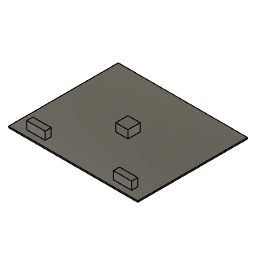
Food_Chain_Magnate_Cover v2 (Autodesk Fusion 360 design; units mm, degrees)
Autodesk Fusion 360 part; units mm, degrees
sketch "Sketch1" plane through (0, 0, 0) normal (0, 0, 1) x (1, 0, 0)
  line L0 (-25, 25) -> (187, 25)
  line L1 (187, 25) -> (187, -155)
  line L2 (187, -155) -> (-25, -155)
  line L3 (-25, -155) -> (-25, 25)
  dimension "d1" = 212
  dimension "d2" = 180
  constraint horizontal L0
  constraint vertical L1
  constraint horizontal L2
  constraint vertical L3
  measures "d1" distance of L0.start L0.end
  measures "d2" distance of L0.start L2.end
extrude "Extrude1" add sketch "Sketch1" along normal blind 2
sketch "Sketch2" plane through (0, 0, 2) normal (0, 0, 1) x (-1, 0, 0)
  line L0 (25, 155) -> (-187, 155)
  line L1 (-187, 155) -> (-187, -25)
  line L2 (-187, -25) -> (25, -25)
  line L3 (25, -25) -> (25, 155)
  line L4 (25, -25) -> (-187, 155) construction
  line L5 (25, 155) -> (-187, -25) construction
  line L6 (25, 65) -> (-81, 65) construction
  line L7 (-187, 65) -> (-81, 65) construction
  line L8 (-81, 65) -> (-81, -25) construction
  line L9 (-81, 65) -> (-81, 155) construction
  line L10 (25, 155) -> (5, 155) construction
  line L11 (5, 155) -> (5, 135) construction
  line L12 (5, 135) -> (25, 135) construction
  line L13 (25, 135) -> (25, 155) construction
  line L14 (-187, 155) -> (-167, 155) construction
  line L15 (-167, 145) -> (-167, 135)
  line L16 (-167, 135) -> (-187, 135) construction
  line L17 (-187, 135) -> (-187, 155) construction
  line L18 (-187, -25) -> (-167, -25) construction
  line L19 (-167, -25) -> (-167, -5) construction
  line L20 (-167, -5) -> (-187, -5) construction
  line L21 (-187, -5) -> (-187, -25) construction
  line L22 (25, -25) -> (5, -25) construction
  line L23 (5, -25) -> (5, -5) construction
  line L24 (5, -5) -> (25, -5) construction
  line L25 (25, -5) -> (25, -25) construction
  line L26 (-167, 135) -> (-137, 135)
  line L27 (-137, 135) -> (-137, 145)
  line L28 (-137, 145) -> (-167, 145)
  line L29 (-167, 145) -> (-167, 135) construction
  line L30 (5, 135) -> (-25, 135)
  line L31 (-25, 135) -> (-25, 145)
  line L32 (-25, 145) -> (5, 145)
  line L33 (5, 145) -> (5, 135)
  line L34 (-167, 155) -> (-167, 145) construction
  line L35 (-71, 55) -> (-91, 55)
  line L36 (-91, 55) -> (-91, 75)
  line L37 (-91, 75) -> (-71, 75)
  line L38 (-71, 75) -> (-71, 55)
  line L39 (-71, 55) -> (-91, 75) construction
  line L40 (-91, 55) -> (-71, 75) construction
  point P0 (-81, 65)
  dimension "d5" = 20
  dimension "d6" = 20
  dimension "d7" = 20
  dimension "d8" = 20
  dimension "d9" = 20
  dimension "d10" = 20
  dimension "d11" = 20
  dimension "d12" = 20
  dimension "d13" = 30
  dimension "d14" = 10
  dimension "d15" = 30
  dimension "d16" = 10
  dimension "d17" = 20
  dimension "d18" = 20
  constraint coincident L2.end L3.start
  constraint coincident L0.end L1.start
  constraint coincident L0.start L3.end
  constraint coincident L1.end L2.start
  constraint midpoint L3 L6.start
  constraint midpoint L5 P0
  constraint midpoint L1 L7.start
  constraint midpoint L2 L8.end
  constraint midpoint L0 L9.end
  constraint horizontal L10
  constraint vertical L11
  constraint horizontal L12
  constraint vertical L13
  constraint horizontal L14
  constraint vertical L15
  constraint horizontal L16
  constraint vertical L17
  constraint horizontal L18
  constraint vertical L19
  constraint horizontal L20
  constraint vertical L21
  constraint horizontal L22
  constraint vertical L23
  constraint horizontal L24
  constraint vertical L25
  constraint horizontal L26
  constraint vertical L27
  constraint horizontal L28
  constraint vertical L29
  constraint horizontal L30
  constraint vertical L31
  constraint horizontal L32
  constraint vertical L33
  constraint perpendicular L28 L34
  constraint horizontal L35
  constraint perpendicular L35 L36
  constraint parallel L35 L37
  constraint parallel L36 L38
  constraint coincident L39 P0
  constraint coincident L40 P0
  constraint coincident P0 L6.end
  measures "d5" distance of L0.start L10.end
  measures "d6" distance of L0.start L12.end
  measures "d7" distance of L0.end L14.end
  measures "d8" distance of L0.end L16.end
  measures "d9" distance of L1.end L18.end
  measures "d10" distance of L1.end L20.end
  measures "d11" distance of L2.end L22.end
  measures "d12" distance of L2.end L24.end
  measures "d13" distance of L15.end L26.end
  measures "d14" distance of L15.end L15.start
  measures "d15" distance of L11.end L30.end
  measures "d16" distance of L11.end L32.end
  measures "d17" distance of L36.end L37.end
  measures "d18" distance of L35.end L36.end
extrude "Extrude2" add sketch "Sketch2" along normal blind 13 contours L15 L26 L27 L28 | L30 L31 L32 L33 | L35 L36 L37 L38
